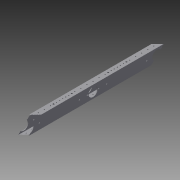
# Autodesk Inventor part: frame_long
Saved by Autodesk Inventor 2015 SP1 (Build 190203100, 203)
## iProperties
Created: 2014-12-21
Part Number: frame_long
Material: Generic
Document SubType Name: Modeling
Designer: Jarod
Density: 1 g/cm^3
Appearance: Default
Author: Jarod
Autodesk Inventor part; units mm, degrees
ref_plane "YZ Plane" through (0, 0, 0) normal (1, 0, 0) x (0, 1, 0)
ref_plane "XZ Plane" through (0, 0, 0) normal (0, 1, 0) x (-1, 0, 0)
ref_plane "XY Plane" through (0, 0, 0) normal (0, 0, 1) x (1, 0, 0)
sketch "Sketch1" plane through (0, 0, 0) normal (0, 0, 1) x (1, 0, 0)
  line L0 (0, 0) -> (25.4, 0)
  line L1 (25.4, 0) -> (25.4, 50.8)
  line L2 (25.4, 50.8) -> (0, 50.8)
  line L3 (0, 50.8) -> (0, 0)
  line L4 (2.54, 2.54) -> (22.86, 2.54)
  line L5 (22.86, 2.54) -> (22.86, 48.26)
  line L6 (22.86, 48.26) -> (2.54, 48.26)
  line L7 (2.54, 48.26) -> (2.54, 2.54)
  dimension "d0" = 25.4
  dimension "d1" = 50.8
  dimension "d2" = 45.72
  dimension "d3" = 20.32
  dimension "d4" = 2.54
  dimension "d5" = 2.54
  constraints: 16 end point, 4 parallel, 2 horizontal, 2 perpendicular
  measures "d0" distance of L2.end L1.end
  measures "d1" distance of L1.end L0.end
  measures "d2" distance of L4.end L5.end
  measures "d3" distance between parallel lines of L5 L7
  measures "d4" distance between parallel lines of L3 L7
  measures "d5" distance between parallel lines of L0 L4
extrude "Extrusion1" add sketch "Sketch1" along normal blind 660.4
sketch "Sketch2" plane through (0, 50.8, 0) normal (0, 1, 0) x (1, 0, 0)
  line L0 (25.4, 0) -> (0, 0) projected
  line L1 (0, 0) -> (0, -660.4) projected
  line L2 (25.4, -660.4) -> (0, -660.4) projected
  line L3 (25.4, 0) -> (25.4, -660.4) projected
  point P0 (12.7, -12.7)
  dimension "d8" = 12.7
  dimension "d9" = 12.7
  measures "d8" distance from line of L3 point (12.7, -12.7)
  measures "d9" distance from line of L0 point (12.7, -12.7)
hole "Hole1" at (12.7, 50.8, 12.7) direction (0, -1, 0) diameter 3.9688 end through all
pattern_linear "Rectangular Pattern1" count 26 spacing 25.4 along (0, 0, 1) of "Hole1"
sketch "Sketch3" plane through (25.4, 0, 0) normal (1, 0, 0) x (0, 0, -1)
  line L0 (0, 0) -> (0, 50.8) projected
  line L1 (0, 50.8) -> (-660.4, 50.8) projected
  line L2 (-660.4, 0) -> (-660.4, 50.8) projected
  line L3 (0, 0) -> (-660.4, 0) projected
  point P0 (-596.9, 25.4)
  point P1 (-330.2, 25.4)
  point P2 (-63.5, 25.4)
  dimension "d20" = 63.5
  dimension "d21" = 25.4
  dimension "d22" = 63.5
  dimension "d23" = 25.4
  dimension "d24" = 25.4
  dimension "d25" = 330.2
  measures "d20" distance from line of L2 point (-596.9, 25.4)
  measures "d21" distance from line of L1 point (-596.9, 25.4)
  measures "d22" distance from line of L0 point (-63.5, 25.4)
  measures "d23" distance from line of L1 point (-63.5, 25.4)
  measures "d24" distance from line of L1 point (-330.2, 25.4)
  measures "d25" distance from line of L2 point (-330.2, 25.4)
hole "Hole2" at (25.4, 25.4, 596.9) at (25.4, 25.4, 330.2) at (25.4, 25.4, 63.5) direction (-1, 0, 0) diameter 38.1 end through all
sketch "Sketch4" plane through (25.4, 0, 0) normal (1, 0, 0) x (0, 0, -1)
  circle A0 centre (-330.2, 25.4) radius 19.05 projected
  circle A1 centre (-596.9, 25.4) radius 19.05 projected
  circle A2 centre (-63.5, 25.4) radius 19.05 projected
  line L0 (0, 0) -> (0, 50.8) projected
  line L1 (0, 50.8) -> (-660.4, 50.8) projected
  line L2 (-660.4, 0) -> (-660.4, 50.8) projected
  line L3 (0, 0) -> (-660.4, 0) projected
  point P0 (-387.35, 25.4)
  point P1 (-273.05, 25.4)
  point P2 (-354.0125, 25.4)
  point P3 (-306.3875, 25.4)
  dimension "d33" = 57.15
  dimension "d34" = 57.15
  dimension "d35" = 25.4
  dimension "d36" = 25.4
  dimension "d37" = 25.4
  dimension "d38" = 25.4
  dimension "d39" = 23.8125
  dimension "d40" = 23.8125
  measures "d33" distance of A0.centre point (-387.35, 25.4)
  measures "d34" distance of A0.centre point (-273.05, 25.4)
  measures "d35" distance from line of L1 point (-273.05, 25.4)
  measures "d36" distance from line of L1 point (-387.35, 25.4)
  measures "d37" distance from line of L1 point (-354.013, 25.4)
  measures "d38" distance from line of L1 point (-306.388, 25.4)
  measures "d39" distance of point (-306.388, 25.4) A0.centre
  measures "d40" distance of A0.centre point (-354.013, 25.4)
hole "Hole3" at (25.4, 25.4, 387.35) at (25.4, 25.4, 273.05) at (25.4, 25.4, 354.0125) at (25.4, 25.4, 306.3875) direction (-1, 0, 0) diameter 4.826 end through all
sketch "Sketch5" plane through (0, 0, 0) normal (-1, 0, 0) x (0, 0, 1)
  circle A0 centre (354.0125, 25.4) radius 2.413 projected
  circle A1 centre (387.35, 25.4) radius 2.413 projected
  circle A2 centre (273.05, 25.4) radius 2.413 projected
  circle A3 centre (306.3875, 25.4) radius 2.413 projected
  circle A4 centre (330.2, 25.4) radius 19.05 projected
  circle A5 centre (596.9, 25.4) radius 19.05 projected
  circle A6 centre (63.5, 25.4) radius 19.05 projected
  line L0 (0, 50.8) -> (0, 0) projected
  line L1 (0, 0) -> (660.4, 0) projected
  line L2 (660.4, 50.8) -> (660.4, 0) projected
  line L3 (0, 50.8) -> (660.4, 50.8) projected
  point P0 (105.5687, 25.4)
  point P1 (554.8313, 25.4)
  dimension "d48" = 25.4
  dimension "d49" = 25.4
  dimension "d50" = 105.5687
  dimension "d51" = 105.5687
  measures "d48" distance from line of L3 point (105.569, 25.4)
  measures "d49" distance from line of L3 point (554.831, 25.4)
  measures "d50" distance from line of L0 point (105.569, 25.4)
  measures "d51" distance from line of point (554.831, 25.4) L2
hole "Hole4" at (0, 25.4, 105.5687) at (0, 25.4, 554.8313) direction (1, 0, 0) diameter 4.826 end through all
sketch "Sketch6" plane through (0, 50.8, 0) normal (0, 1, 0) x (1, 0, 0)
  circle A0 centre (12.7, -647.7) radius 1.9844 projected
  circle A1 centre (12.7, -622.3) radius 1.9844 projected
  circle A2 centre (12.7, -596.9) radius 1.9844 projected
  circle A3 centre (12.7, -571.5) radius 1.9844 projected
  circle A4 centre (12.7, -546.1) radius 1.9844 projected
  circle A5 centre (12.7, -520.7) radius 1.9844 projected
  circle A6 centre (12.7, -495.3) radius 1.9844 projected
  circle A7 centre (12.7, -469.9) radius 1.9844 projected
  circle A8 centre (12.7, -444.5) radius 1.9844 projected
  circle A9 centre (12.7, -419.1) radius 1.9844 projected
  circle A10 centre (12.7, -393.7) radius 1.9844 projected
  circle A11 centre (12.7, -368.3) radius 1.9844 projected
  circle A12 centre (12.7, -342.9) radius 1.9844 projected
  circle A13 centre (12.7, -317.5) radius 1.9844 projected
  circle A14 centre (12.7, -292.1) radius 1.9844 projected
  circle A15 centre (12.7, -266.7) radius 1.9844 projected
  circle A16 centre (12.7, -241.3) radius 1.9844 projected
  circle A17 centre (12.7, -215.9) radius 1.9844 projected
  circle A18 centre (12.7, -190.5) radius 1.9844 projected
  circle A19 centre (12.7, -165.1) radius 1.9844 projected
  circle A20 centre (12.7, -139.7) radius 1.9844 projected
  circle A21 centre (12.7, -114.3) radius 1.9844 projected
  circle A22 centre (12.7, -88.9) radius 1.9844 projected
  circle A23 centre (12.7, -63.5) radius 1.9844 projected
  circle A24 centre (12.7, -38.1) radius 1.9844 projected
  circle A25 centre (12.7, -12.7) radius 1.9844 projected
  line L0 (25.4, 0) -> (0, 0) projected
  line L1 (0, 0) -> (0, -660.4) projected
  line L2 (25.4, -660.4) -> (0, -660.4) projected
  line L3 (25.4, 0) -> (25.4, -660.4) projected
  circle A26 centre (12.7, -647.7) radius 1.9844 projected
  circle A27 centre (12.7, -647.7) radius 3.175
  circle A28 centre (12.7, -12.7) radius 3.175
  circle A29 centre (12.7, -25.4) radius 3.175
  circle A30 centre (12.7, -635) radius 3.175
  dimension "d59" = 6.35
  dimension "d60" = 6.35
  dimension "d61" = 25.4
  dimension "d62" = 12.7
  dimension "d63" = 6.35
  dimension "d64" = 25.4
  dimension "d65" = 12.7
  dimension "d66" = 6.35
  constraints: 4 centre point, 4 coincident
  measures "d59" diameter of A27
  measures "d60" diameter of A28
  measures "d61" distance from line of L0 point (12.7, -25.4)
  measures "d62" distance from line of L3 point (12.7, -25.4)
  measures "d63" diameter of A29
  measures "d64" distance from line of L2 point (12.7, -635)
  measures "d65" distance from line of L3 point (12.7, -635)
  measures "d66" diameter of A30
extrude "Extrusion2" cut sketch "Sketch6" against normal blind 50.8 contours A27 | A28 | A29 | A30
sketch "Sketch7" plane through (0, 50.8, 0) normal (0, 1, 0) x (1, 0, 0)
  circle A0 centre (12.7, -25.4) radius 3.175 projected
  circle A1 centre (12.7, -647.7) radius 3.175 projected
  circle A2 centre (12.7, -12.7) radius 3.175 projected
  circle A3 centre (12.7, -635) radius 3.175 projected
  circle A4 centre (12.7, -622.3) radius 1.9844 projected
  circle A5 centre (12.7, -596.9) radius 1.9844 projected
  circle A6 centre (12.7, -571.5) radius 1.9844 projected
  circle A7 centre (12.7, -546.1) radius 1.9844 projected
  circle A8 centre (12.7, -520.7) radius 1.9844 projected
  circle A9 centre (12.7, -495.3) radius 1.9844 projected
  circle A10 centre (12.7, -469.9) radius 1.9844 projected
  circle A11 centre (12.7, -444.5) radius 1.9844 projected
  circle A12 centre (12.7, -419.1) radius 1.9844 projected
  circle A13 centre (12.7, -393.7) radius 1.9844 projected
  circle A14 centre (12.7, -368.3) radius 1.9844 projected
  circle A15 centre (12.7, -342.9) radius 1.9844 projected
  circle A16 centre (12.7, -317.5) radius 1.9844 projected
  circle A17 centre (12.7, -292.1) radius 1.9844 projected
  circle A18 centre (12.7, -266.7) radius 1.9844 projected
  circle A19 centre (12.7, -241.3) radius 1.9844 projected
  circle A20 centre (12.7, -215.9) radius 1.9844 projected
  circle A21 centre (12.7, -190.5) radius 1.9844 projected
  circle A22 centre (12.7, -165.1) radius 1.9844 projected
  circle A23 centre (12.7, -139.7) radius 1.9844 projected
  circle A24 centre (12.7, -114.3) radius 1.9844 projected
  circle A25 centre (12.7, -88.9) radius 1.9844 projected
  circle A26 centre (12.7, -63.5) radius 1.9844 projected
  circle A27 centre (12.7, -38.1) radius 1.9844 projected
  line L0 (25.4, 0) -> (0, 0) projected
  line L1 (0, 0) -> (0, -660.4) projected
  line L2 (25.4, -660.4) -> (0, -660.4) projected
  line L3 (25.4, 0) -> (25.4, -660.4) projected
  point P0 (12.7, -482.6)
  point P1 (12.7, -457.2)
  point P2 (12.7, -431.8)
  point P3 (12.7, -406.4)
  point P4 (12.7, -254)
  point P5 (12.7, -228.6)
  point P6 (12.7, -203.2)
  point P7 (12.7, -177.8)
  dimension "d69" = 177.8
  dimension "d70" = 203.2
  dimension "d71" = 228.6
  dimension "d72" = 254
  dimension "d73" = 12.7
  dimension "d74" = 12.7
  dimension "d75" = 12.7
  dimension "d76" = 12.7
  dimension "d77" = 12.7
  dimension "d78" = 12.7
  dimension "d79" = 12.7
  dimension "d80" = 12.7
  dimension "d81" = 177.8
  dimension "d82" = 203.2
  dimension "d83" = 228.6
  dimension "d84" = 254
  measures "d69" vertical distance of L2.start point (12.7, -482.6)
  measures "d70" vertical distance of L2.start point (12.7, -457.2)
  measures "d71" vertical distance of L2.start point (12.7, -431.8)
  measures "d72" vertical distance of L2.start point (12.7, -406.4)
  measures "d73" distance from line of L3 point (12.7, -482.6)
  measures "d74" distance from line of L3 point (12.7, -457.2)
  measures "d75" distance from line of L3 point (12.7, -431.8)
  measures "d76" distance from line of L3 point (12.7, -406.4)
  measures "d77" distance from line of L3 point (12.7, -177.8)
  measures "d78" distance from line of L3 point (12.7, -203.2)
  measures "d79" distance from line of L3 point (12.7, -228.6)
  measures "d80" distance from line of L3 point (12.7, -254)
  measures "d81" distance from line of point (12.7, -177.8) L0
  measures "d82" distance from line of point (12.7, -203.2) L0
  measures "d83" distance from line of point (12.7, -228.6) L0
  measures "d84" distance from line of point (12.7, -254) L0
hole "Hole5" at (12.7, 50.8, 482.6) at (12.7, 50.8, 457.2) at (12.7, 50.8, 431.8) at (12.7, 50.8, 406.4) at (12.7, 50.8, 254) at (12.7, 50.8, 228.6) at (12.7, 50.8, 203.2) at (12.7, 50.8, 177.8) direction (0, -1, 0) diameter 3.9688 end through all
sketch "Sketch8" plane through (0, 50.8, 0) normal (0, 1, 0) x (1, 0, 0)
  circle A0 centre (12.7, -203.2) radius 1.9844 projected
  circle A1 centre (12.7, -254) radius 1.9844 projected
  circle A2 centre (12.7, -431.8) radius 1.9844 projected
  circle A3 centre (12.7, -482.6) radius 1.9844 projected
  circle A4 centre (12.7, -457.2) radius 1.9844 projected
  circle A5 centre (12.7, -406.4) radius 1.9844 projected
  circle A6 centre (12.7, -228.6) radius 1.9844 projected
  circle A7 centre (12.7, -177.8) radius 1.9844 projected
  circle A8 centre (12.7, -25.4) radius 3.175 projected
  circle A9 centre (12.7, -647.7) radius 3.175 projected
  circle A10 centre (12.7, -12.7) radius 3.175 projected
  circle A11 centre (12.7, -635) radius 3.175 projected
  circle A12 centre (12.7, -622.3) radius 1.9844 projected
  circle A13 centre (12.7, -596.9) radius 1.9844 projected
  circle A14 centre (12.7, -571.5) radius 1.9844 projected
  circle A15 centre (12.7, -546.1) radius 1.9844 projected
  circle A16 centre (12.7, -520.7) radius 1.9844 projected
  circle A17 centre (12.7, -495.3) radius 1.9844 projected
  circle A18 centre (12.7, -469.9) radius 1.9844 projected
  circle A19 centre (12.7, -444.5) radius 1.9844 projected
  circle A20 centre (12.7, -419.1) radius 1.9844 projected
  circle A21 centre (12.7, -393.7) radius 1.9844 projected
  circle A22 centre (12.7, -368.3) radius 1.9844 projected
  circle A23 centre (12.7, -342.9) radius 1.9844 projected
  circle A24 centre (12.7, -317.5) radius 1.9844 projected
  circle A25 centre (12.7, -292.1) radius 1.9844 projected
  circle A26 centre (12.7, -266.7) radius 1.9844 projected
  circle A27 centre (12.7, -241.3) radius 1.9844 projected
  circle A28 centre (12.7, -215.9) radius 1.9844 projected
  circle A29 centre (12.7, -190.5) radius 1.9844 projected
  circle A30 centre (12.7, -165.1) radius 1.9844 projected
  circle A31 centre (12.7, -139.7) radius 1.9844 projected
  circle A32 centre (12.7, -114.3) radius 1.9844 projected
  circle A33 centre (12.7, -88.9) radius 1.9844 projected
  circle A34 centre (12.7, -63.5) radius 1.9844 projected
  circle A35 centre (12.7, -38.1) radius 1.9844 projected
  line L0 (25.4, 0) -> (0, 0) projected
  line L1 (0, 0) -> (0, -660.4) projected
  line L2 (25.4, -660.4) -> (0, -660.4) projected
  line L3 (25.4, 0) -> (25.4, -660.4) projected
  circle A36 centre (12.7, -482.6) radius 3.175
  circle A37 centre (12.7, -406.4) radius 3.175
  circle A38 centre (12.7, -254) radius 3.175
  circle A39 centre (12.7, -177.8) radius 3.175
  dimension "d92" = 6.35
  dimension "d93" = 6.35
  dimension "d94" = 6.35
  dimension "d95" = 6.35
  constraints: 4 centre point, 4 coincident
  measures "d92" diameter of A36
  measures "d93" diameter of A37
  measures "d94" diameter of A38
  measures "d95" diameter of A39
extrude "Extrusion3" cut sketch "Sketch8" against normal blind 50.8 contours A36 | A37 | A38 | A39
body "Solid1"
